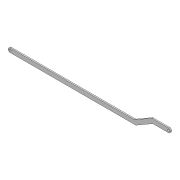
# Autodesk Inventor part: FRC001-1
Saved by Autodesk Inventor 2020 (Build 240168000, 168)
## iProperties
Created: 2020-02-18
Part Number: FRC001-1
Material: Generic
Document SubType Name: Modeling
Designer: Juan carlos Botero
Density: 1 g/cm^3
Appearance: Default
Mass: 96.6859 g
Surface Area: 425.54 cm^2
Volume: 96.6859 cm^3
Engineer: Juan carlos Botero
Authority: Jorge Barrera
Author: Juan carlos Botero
Title: BARRA
Autodesk Inventor part; units mm, degrees
ref_plane "YZ Plane" through (0, 0, 0) normal (1, 0, 0) x (0, 1, 0)
ref_plane "XZ Plane" through (0, 0, 0) normal (0, 1, 0) x (-1, 0, 0)
ref_plane "XY Plane" through (0, 0, 0) normal (0, 0, 1) x (1, 0, 0)
sketch "Sketch1" plane through (0, 0, 0) normal (0, 0, 1) x (1, 0, 0)
  circle A0 centre (775, 48) radius 5
  circle A1 centre (0, 0) radius 5
  line L0 (0, 0) -> (611.8616, 0) construction
  line L1 (0, -10) -> (611.8616, -10)
  line L2 (611.8616, 10) -> (0, 10)
  arc A2 (0, 10) -> (0, -10) centre (0, 0) ccw
  arc A3 (611.8616, -10) -> (611.8616, 10) centre (611.8616, 0) ccw
  line L3 (611.8616, 0) -> (695, 48) construction
  line L4 (616.8616, -8.6603) -> (700, 39.3397)
  line L5 (690, 56.6603) -> (606.8616, 8.6603)
  arc A4 (606.8616, 8.6603) -> (616.8616, -8.6603) centre (611.8616, 0) ccw
  arc A5 (700, 39.3397) -> (690, 56.6603) centre (695, 48) ccw
  line L6 (695, 48) -> (775, 48) construction
  line L7 (695, 38) -> (775, 38)
  line L8 (775, 58) -> (695, 58)
  arc A6 (695, 58) -> (695, 38) centre (695, 48) ccw
  arc A7 (775, 38) -> (775, 58) centre (775, 48) ccw
  point P0 (305.9308, 0)
  point P1 (653.4308, 24)
  point P2 (735, 48)
  point P3 (616.8616, -8.6603)
  point P4 (697.6795, 38)
  point P5 (609.1821, 10)
  dimension "d0" = 775
  dimension "d1" = 10
  dimension "d2" = 48
  dimension "d4" = 10
  dimension "d5" = 30
  dimension "d6" = 80
  constraints: 24 end point, 12 point on circle, 12 tangent, 8 centre point, 4 parallel, 3 equal radius, 3 midpoint, 1 coincident, 1 horizontal
  measures "d0" horizontal distance of L6.end point (0, 0)
  measures "d1" diameter of A1
  measures "d2" vertical distance of point (0, 0) L6.end
  measures "d4" radius of A2
  measures "d5" angle of L0 L3
  measures "d6" distance of L3.end L6.end
extrude "Extrusion1" add sketch "Sketch1" along normal blind 6
fillet "Fillet1" radius 10 2 edges at (697.6795, 38, 3) (609.1821, 10, 3)
body "Solid1"
